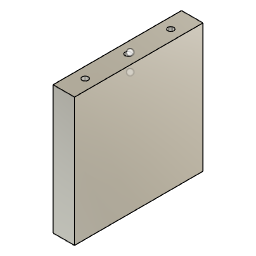
securing_structure_wall v15 (Autodesk Fusion 360 design; units mm, degrees)
Autodesk Fusion 360 part; units mm, degrees
note: some values were not read from the file. Chosen so that the rebuilt part matches the saved one: which bodies a step acts on; which face or edge a step refers to; how an offset face is resized; which pieces of a blend or face edit are solid.
sketch "Sketch1" plane through (0, 0, 0) normal (1, 0, 0) x (0, 1, 0)
  line L0 (0, 0) -> (150, 0)
  line L1 (150, 0) -> (150, 152.719)
  line L2 (150, 152.719) -> (0, 152.719)
  line L3 (0, 152.719) -> (0, 0)
  dimension "d1_1" = 150
  dimension "d2_1" = 152.719
  constraint horizontal L0
  constraint vertical L1
  constraint horizontal L2
  constraint vertical L3
  constraint coincident L0.start L3.end
  measures "d1_1" distance of L0.start L0.end
  measures "d2_1" distance of L0.start L2.end
extrude "Extrude1" add sketch "Sketch1" along normal blind 20 makes body 1
sketch "Sketch2" plane through (20, 0, 0) normal (1, 0, 0) x (0, 1, 0)
  line L0 (0, 152.719) -> (0, 0)
  line L1 (0, 0) -> (150, 0)
  line L2 (150, 0) -> (150, 152.719)
  line L3 (150, 152.719) -> (0, 152.719)
  line L4 (75, 152.719) -> (46.5, 152.719)
  line L5 (75, 152.719) -> (103.5, 152.719)
  line L6 (103.5, 152.719) -> (46.5, 152.719)
  line L7 (46.5, 152.719) -> (46.5, 142.719)
  line L8 (46.5, 142.719) -> (103.5, 142.719)
  line L9 (103.5, 142.719) -> (103.5, 152.719)
  dimension "d5_1" = 28.5
  dimension "d6_1" = 28.5
  dimension "d7_1" = 57
  dimension "d8_1" = 10
  constraint midpoint L3 L4.start
  constraint parallel L3 L4
  constraint parallel L3 L5
  constraint horizontal L6
  constraint vertical L7
  constraint horizontal L8
  constraint vertical L9
  measures "d5_1" distance of L4.start L4.end
  measures "d6_1" distance of L4.start L5.end
  measures "d7_1" distance of L5.end L4.end
  measures "d8_1" distance of L5.end L8.end
extrude "Extrude2" cut sketch "Sketch2" against normal blind 70 contours L3 L4 L5 L6 L7 L8 L9 bodies 1
extrude "Extrude3" cut 1 faces at (13.3333, 65.5, 142.719) along direction (0, 0, -1) blind 10 on bodies 1 bodies 1
extrude "Extrude4" cut 2 faces at (6.6667, 31, 152.719) (6.6667, 134.5, 152.719) along direction (0, 0, -1) blind 20 on bodies 1 bodies 1
sketch "Sketch3" plane through (0, 0, 132.719) normal (0, 0, 1) x (-1, 0, 0)
  line L0 (0, -150) -> (0, 0)
  line L1 (0, 0) -> (-20, 0)
  line L2 (-20, 0) -> (-20, -150)
  line L3 (-20, -150) -> (0, -150)
  line L4 (-10, 0) -> (-10, -25)
  line L5 (-10, -150) -> (-10, -125)
  line L6 (-10, -125) -> (-10, -75)
  dimension "d15_1" = 25
  dimension "d16_1" = 25
  constraint midpoint L1 L4.start
  constraint perpendicular L1 L4
  constraint midpoint L3 L5.start
  constraint perpendicular L3 L5
  constraint parallel L5 L6
  measures "d15_1" distance of L4.start L4.end
  measures "d16_1" distance of L5.start L5.end
hole "Hole1" at (10, 75, 132.719) at (10, 125, 132.719) at (10, 25, 132.719) direction (0, 0, -1) diameter 7.035 depth 10 tip angle 180 bodies 1
thread "Thread1" "ISO Metric profile 8.0 M8x1 6H"
sketch "Sketch4" plane through (0, 0, 0) normal (0, 0, -1) x (1, 0, 0)
  line L0 (0, 0) -> (0, -150)
  line L1 (0, -150) -> (20, -150)
  line L2 (20, -150) -> (20, 0)
  line L3 (20, 0) -> (0, 0)
  line L4 (10, -150) -> (10, -125)
  line L5 (10, 0) -> (10, -25)
  line L6 (10, -75) -> (10, -25)
  dimension "d20_1" = 25
  dimension "d21_1" = 25
  constraint midpoint L1 L4.start
  constraint perpendicular L1 L4
  constraint midpoint L3 L5.start
  constraint perpendicular L3 L5
  constraint parallel L5 L6
  measures "d20_1" distance of L4.start L4.end
  measures "d21_1" distance of L5.start L5.end
delete_face "DeleteFace1" 2 faces at (10.1753, 71.4869, 129.3857) (10.8869, 73.5611, 122.719) on bodies 1
hole "Hole3" at (10, 75, 132.719) direction (0, 0, -1) diameter 7.035 depth 10 tip angle 180 bodies 1
thread "Thread3" "ISO Metric profile 8.0 M8x1 6H"
hole "Hole4" at (10, 75, 152.719) direction (0, 0, -1) diameter 6.78 depth 80 tip angle 180 bodies 1
delete_face "DeleteFace2" 1 faces at (10.169, 71.6142, 106.0523) on bodies 1
extrude "Extrude5" add 1 faces at (10, 142.8392, 132.719) along direction (0, 0, 1) blind 13 on bodies 1 bodies 1
extrude "Extrude6" add 3 faces at (7.7223, 125.9756, 122.719) (10.8869, 73.5611, 122.719) (10.8869, 23.5611, 122.719) along direction (0, 0, 1) blind 13 on bodies 1 bodies 1
extrude "Extrude7" add 1 faces at (0, 71.2392, 24.2397) along direction (-1, 0, 0) blind 5 on bodies 1 bodies 1
sketch "Sketch5" plane through (0, 0, 0) normal (0, 0, -1) x (1, 0, 0)
  line L0 (-5, -150) -> (20, -150)
  line L1 (20, -150) -> (20, 0)
  line L2 (20, 0) -> (-5, 0)
  line L3 (-5, 0) -> (-5, -150)
  line L4 (7.5, 0) -> (7.5, -25)
  line L5 (7.5, -150) -> (7.5, -125)
  line L6 (7.5, -125) -> (7.5, -75)
  dimension "d31" = 25
  dimension "d32" = 25
  dimension "d33" = 50
  constraint midpoint L2 L4.start
  constraint perpendicular L2 L4
  constraint midpoint L0 L5.start
  constraint perpendicular L0 L5
  constraint parallel L5 L6
  measures "d31" distance of L4.start L4.end
  measures "d32" distance of L5.start L5.end
  measures "d33" distance of L5.end L6.end
hole "Hole5" at (7.5, 25, 0) at (7.5, 75, 0) at (7.5, 125, 0) direction (0, 0, 1) diameter 6.78 depth 20 tip angle 180 bodies 1
thread "Thread5" "ISO Metric profile 8.0 M8x1 6H" major diameter 8.147 minor diameter 7.035 pitch 1 angle 60 resizes the face on face at (7.669, 28.3858, 6.6667) on face at (7.669, 78.3858, 6.6667) on face at (5.8787, 127.9772, 13.3333) on bodies 1
delete_face "DeleteFace3" 2 faces at (10.3502, 121.5, 139.0523) (7.7223, 125.9756, 135.719) on bodies 1
delete_face "DeleteFace4" 2 faces at (10.3502, 71.5, 139.0523) (10.8869, 73.5611, 135.719) on bodies 1
delete_face "DeleteFace5" 1 faces at (10.3502, 21.5, 139.0523) on bodies 1
sketch "Sketch6" plane through (0, 0, 145.719) normal (0, 0, 1) x (-1, 0, 0)
  line L0 (5, 0) -> (-20, 0)
  line L1 (-20, 0) -> (-20, -150)
  line L2 (-20, -150) -> (5, -150)
  line L3 (5, -150) -> (5, 0)
  line L4 (-7.5, 0) -> (-7.5, -25)
  line L5 (-7.5, -25) -> (-7.5, -75)
  line L6 (-7.5, -150) -> (-7.5, -125)
  dimension "d37" = 25
  dimension "d38" = 50
  dimension "d39" = 25
  constraint midpoint L0 L4.start
  constraint perpendicular L0 L4
  constraint parallel L4 L5
  constraint midpoint L2 L6.start
  constraint perpendicular L2 L6
  measures "d37" distance of L4.start L4.end
  measures "d38" distance of L4.end L5.end
  measures "d39" distance of L6.start L6.end
hole "Hole6" at (7.5, 125, 145.719) at (7.5, 75, 145.719) at (7.5, 25, 145.719) direction (0, 0, -1) diameter 6.78 depth 20 tip angle 180 bodies 1
thread "Thread6" "ISO Metric profile 8.0 M8x1 6H" major diameter 8.147 minor diameter 7.035 pitch 1 angle 60 resizes the face on face at (7.669, 121.6142, 139.0523) on face at (7.669, 71.6142, 139.0523) on face at (7.669, 21.6142, 139.0523) on bodies 1
ref_plane "WorkPlane1" through (7.5, 75, 85.719) normal (0, 0, 1) x (1, 0, 0)
split "Split1" by plane through (7.5, 75, 85.719) normal (0, 0, 1) bodies 1 makes body 2 at (20, 100, 105.719)
move_body "Move1" bodies 2 to x (1, 0, 0) y (0, 1, 0) z (0, 0, 1) at (0, 0, 2)
extrude "Extrude8" add 1 faces at (11.6667, 50, 85.719) along direction (0, 0, 1) blind 2 on bodies 1 bodies 1 2
ref_plane "WorkPlane2" through (7.5, 75, 87.719) normal (0, 0, 1) x (1, 0, 0)
split "Split2" by plane through (7.5, 75, 87.719) normal (0, 0, 1) bodies 1 makes body 3 at (20, 50, 127.719)
move_body "Move2" bodies 3 to x (1, 0, 0) y (0, 1, 0) z (0, 0, 1) at (0, 0, 2.711)
extrude "Extrude9" add 1 faces at (11.6667, 50, 87.719) along direction (0, 0, 1) blind 2.281 on bodies 1 bodies 1
move_body "Move3" bodies 3 to x (1, 0, 0) y (0, 1, 0) z (0, 0, 1) at (0, 0, -0.43)
combine "Combine1" operation add target body 1 tool bodies 3
equation "d5_1 = ( 57 / 2 ) * 1 mm"
equation "d6_1 = ( 57 / 2 ) * 1 mm"
